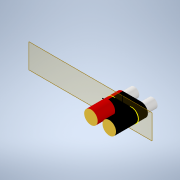
# Autodesk Inventor part: banana plug
Saved by Autodesk Inventor 2022 (Build 260153000, 153)
## iProperties
Created: 2024-07-07
Part Number: banana plug
Material: Типовые
Document SubType Name: Modeling
Designer: Капустяник Андрей
Density: 1 g/cm^3
Appearance: По умолчанию
Author: Капустяник Андрей
Autodesk Inventor part; units mm, degrees
ref_plane "YZ Plane" through (0, 0, 0) normal (1, 0, 0) x (0, 1, 0)
ref_plane "XZ Plane" through (0, 0, 0) normal (0, 1, 0) x (-1, 0, 0)
ref_plane "XY Plane" through (0, 0, 0) normal (0, 0, 1) x (1, 0, 0)
sketch "Эскиз1" plane through (0, 0, 0) normal (0, 0, 1) x (1, 0, 0)
  circle A0 centre (-9.5, 0) radius 7
  circle A1 centre (9.5, 0) radius 7
  line L0 (16.5, 0) -> (-16.5, 0)
  line L1 (9.5, -7) -> (-9.5, -7)
  line L2 (9.5, 7) -> (-9.5, 7)
  point P0 (0, 0)
  point P1 (0, 0)
  dimension "d0" = 14
  dimension "d1" = 14
  dimension "d2" = 33
  constraints: 6 end point, 6 point on circle, 4 tangent, 2 centre point, 2 point on line, 1 coincident, 1 horizontal, 1 midpoint
  measures "d0" diameter of A0
  measures "d1" diameter of A1
  measures "d2" distance of L0.start L0.end
extrude "Выдавливание1" add sketch "Эскиз1" along normal blind 5 and the other way blind 10
sketch "Эскиз2" plane through (0, 0, 5) normal (0, 0, 1) x (1, 0, 0)
  arc A0 (9.5, -7) -> (9.5, 7) centre (9.5, 0) ccw projected
  circle A1 centre (9.5, 0) radius 7
  arc A2 (-9.5, 7) -> (-9.5, -7) centre (-9.5, 0) ccw projected
  circle A3 centre (-9.5, 0) radius 7
  point P0 (0, 0)
  point P1 (-9.5, -7)
  constraints: 2 coincident, 6 other
extrude "Выдавливание2" add sketch "Эскиз2" along normal blind 18
sketch "Эскиз3" plane through (0, 0, -10) normal (0, 0, -1) x (-1, 0, 0)
  arc A0 (9.5, -7) -> (9.5, 7) centre (9.5, 0) ccw projected
  circle A1 centre (9.5, 0) radius 5
  arc A2 (-9.5, 7) -> (-9.5, -7) centre (-9.5, 0) ccw projected
  circle A3 centre (-9.5, 0) radius 5
  point P0 (0, 0)
  dimension "d9" = 10
  dimension "d10" = 10
  constraints: 2 centre point, 2 coincident
  measures "d9" diameter of A1
  measures "d10" diameter of A3
extrude "Выдавливание3" add sketch "Эскиз3" along normal blind 12
ref_plane "РабПлоскость1" through (-90.9653, 8.5, 0) normal (0, 0, 1) x (1, 0, 0)
sketch "Эскиз4" plane through (-90.9653, 8.5, 0) normal (0, 0, 1) x (1, 0, 0)
  circle A0 centre (100.4653, -8.5) radius 7 projected
  circle A1 centre (81.4653, -8.5) radius 7 projected
  arc A2 (100.4653, -15.5) -> (100.4653, -1.5) centre (100.4653, -8.5) ccw projected
  arc A3 (81.4653, -1.5) -> (81.4653, -15.5) centre (81.4653, -8.5) ccw projected
  line L0 (100.4653, -8.5) -> (81.4653, -8.5)
  line L1 (90.9653, -8.5) -> (90.9653, 7)
  line L2 (90.9653, -8.5) -> (70, -8.5)
  constraints: 6 end point, 2 horizontal, 1 coincident, 1 vertical
